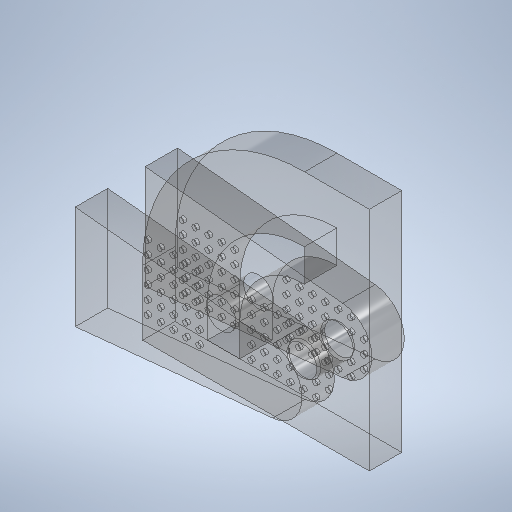
# Autodesk Inventor part: PruebadesoportesmecanismoV1
Saved by Autodesk Inventor 2025.2 (Build 292293000, 293)
## iProperties
Created: 2025-03-25
Part Number: PruebadesoportesmecanismoV1
Material: PVC, no plastificado
Document SubType Name: Modeling
Designer: braug
Density: 1.29 g/cm^3
Appearance: Agua Burbujas
Author: braug
## iProperties of the stored document Prueba de soportes mecanismo_3DPrint.ipt
Created: 2025-03-25
Part Number: Prueba de soportes mecanismo_3DPrint
Material: Genérico
Document SubType Name: Modeling
Designer: braug
Density: 1 g/cm^3
Appearance: Valor por defecto
Author: braug
Autodesk Inventor part; units mm, degrees
ref_plane "YZ Plane" through (0, 0, 0) normal (1, 0, 0) x (0, 1, 0)
ref_plane "XZ Plane" through (0, 0, 0) normal (0, 1, 0) x (-1, 0, 0)
ref_plane "XY Plane" through (0, 0, 0) normal (0, 0, 1) x (1, 0, 0)
sketch "Boceto1" plane through (0, 0, 0) normal (0, 0, 1) x (1, 0, 0)
  line L0 (-35, 0) -> (15, 0)
  line L1 (-20, 10) -> (-20, 0)
  arc A0 (-10, 20) -> (-20, 10) centre (-10, 10) ccw
  arc A1 (-10, 25) -> (-25, 10) centre (-10, 10) ccw
  line L2 (-25, 10) -> (-25, 0)
  arc A2 (-10, 35) -> (-35, 10) centre (-10, 10) ccw
  line L3 (-35, 10) -> (-35, 0)
  line L4 (-35, 0) -> (-10, 0)
  circle A3 centre (-10, 10) radius 2.5
  line L5 (-10, 20) -> (0, 20)
  line L6 (0, 20) -> (0, 21.1803)
  line L7 (0, 25) -> (-10, 25)
  line L8 (-10, 35) -> (0, 35)
  line L9 (0, 35) -> (0, 25)
  line L10 (0, 20) -> (0, 0)
  line L11 (0, 0) -> (-10, 0)
  line L12 (0, 25) -> (0, 20)
  line L13 (-10, 25) -> (-10, 20)
  line L14 (-20, 5) -> (-25, 5)
  point P0 (0, 0)
  dimension "d0" = 20
  dimension "d1" = 25
  dimension "d2" = 10
  dimension "d3" = 10
  dimension "d4" = 5
  dimension "d6" = 35
  constraints: 30 end point, 7 point on circle, 5 point on line, 4 centre point, 3 coincident, 3 collinear, 3 midpoint, 3 perpendicular, 3 tangent, 2 parallel, 1 horizontal
  measures "d0" distance of L5.start L11.end
  measures "d1" distance of L7.end L11.end
  measures "d2" distance of L3.start L0.start
  measures "d3" distance of L11.end A2.centre
  measures "d4" diameter of A3
  measures "d6" distance of L10.end L8.end
extrude "Extrusión1" add sketch "Boceto1" along normal mid plane 5 contours L3 A2 L8 L9 L7 A1 L2 L0 | L2 L14 L1 L0 | L1 A0 L5 L10 L0 | L7 L12 L6 L5 L13
sketch "Boceto2" plane through (0, 0, 2.5) normal (0, 0, 1) x (1, 0, 0)
  circle A0 centre (-10, 10) radius 2.3
  circle A1 centre (-22.5, 10) radius 2.3
  circle A2 centre (-10, 10) radius 2.5 projected
  point P0 (0, 0)
  dimension "d9" = 4.6
  dimension "d10" = 4.6
  constraints: 2 centre point
  measures "d9" diameter of A0
  measures "d10" diameter of A1
extrude "Extrusión2" add sketch "Boceto2" along normal blind 0.4 and the other way blind 5.4 contours A0 | A1
sketch "Boceto3" plane through (-10, 10, 2.9) normal (0, 0, 1) x (1, 0, 0)
  arc A0 (5, 0) -> (0.4927, 4.9757) centre (0, 0) ccw
  line L0 (-30, 0) -> (-30, 7.9951)
  line L1 (0.4927, 4.9757) -> (-30, 7.9951)
  line L2 (-30, 0) -> (-30, -7.9951)
  line L3 (0.4927, -4.9757) -> (-30, -7.9951)
  arc A1 (0.4927, -4.9757) -> (5, 0) centre (0, 0) ccw
  circle A2 centre (0, 0) radius 2.3 projected
  point P0 (10, -10)
  dimension "d15" = 10
  constraints: 8 end point, 4 point on circle, 2 centre point
  measures "d15" diameter of A0
extrude "Extrusión3" add sketch "Boceto3" along normal blind 5 contours A1 L3 L2 L0 L1 A0 | A2
sketch "Boceto4" plane through (-22.5, 10, -2.9) normal (0, 0, -1) x (-1, 0, 0)
  circle A0 centre (0, 0) radius 2.3 projected
  circle A1 centre (-12.5, 0) radius 2.3 projected
  line L0 (-12.9927, 4.9757) -> (17.5, 7.9951) projected
  arc A2 (-12.9927, 4.9757) -> (-12.9927, -4.9757) centre (-12.5, 0) ccw projected
  line L1 (17.5, -7.9951) -> (-12.9927, -4.9757) projected
  line L2 (17.5, 7.9951) -> (17.5, -7.9951) projected
  point P0 (-22.5, -10)
extrude "Extrusión4" add sketch "Boceto4" along normal blind 5 contours A0 | A1 | L0 L2 L1 A2
sketch "Boceto5" plane through (0, 0, -2.5) normal (0, 0, -1) x (-1, 0, 0)
  circle A0 centre (10, 10) radius 2.3 projected
  circle A1 centre (10, 10) radius 0.4
  line L0 (10, 10) -> (10, 1.6419)
  line L1 (10, 1.6419) -> (12.8355, 1.6419)
  circle A2 centre (10, 8) radius 0.4
  circle A3 centre (10, 6) radius 0.4
  circle A4 centre (12, 10) radius 0.4
  circle A5 centre (12, 8) radius 0.4
  circle A6 centre (12, 6) radius 0.4
  circle A7 centre (14, 10) radius 0.4
  circle A8 centre (14, 8) radius 0.4
  circle A9 centre (14, 6) radius 0.4
  circle A10 centre (16, 10) radius 0.4
  circle A11 centre (16, 8) radius 0.4
  circle A12 centre (16, 6) radius 0.4
  circle A13 centre (18, 10) radius 0.4
  circle A14 centre (18, 8) radius 0.4
  circle A15 centre (18, 6) radius 0.4
  circle A16 centre (20, 10) radius 0.4
  circle A17 centre (20, 8) radius 0.4
  circle A18 centre (20, 6) radius 0.4
  circle A19 centre (22, 10) radius 0.4
  circle A20 centre (22, 8) radius 0.4
  circle A21 centre (22, 6) radius 0.4
  circle A22 centre (24, 10) radius 0.4
  circle A23 centre (24, 8) radius 0.4
  circle A24 centre (24, 6) radius 0.4
  circle A25 centre (26, 10) radius 0.4
  circle A26 centre (26, 8) radius 0.4
  circle A27 centre (26, 6) radius 0.4
  circle A28 centre (28, 10) radius 0.4
  circle A29 centre (28, 8) radius 0.4
  circle A30 centre (28, 6) radius 0.4
  circle A31 centre (30, 10) radius 0.4
  circle A32 centre (30, 8) radius 0.4
  circle A33 centre (30, 6) radius 0.4
  circle A34 centre (32, 10) radius 0.4
  circle A35 centre (32, 8) radius 0.4
  circle A36 centre (32, 6) radius 0.4
  circle A37 centre (34, 10) radius 0.4
  circle A38 centre (34, 8) radius 0.4
  circle A39 centre (34, 6) radius 0.4
  circle A40 centre (36, 10) radius 0.4
  circle A41 centre (36, 8) radius 0.4
  circle A42 centre (36, 6) radius 0.4
  circle A43 centre (38, 10) radius 0.4
  circle A44 centre (38, 8) radius 0.4
  circle A45 centre (38, 6) radius 0.4
  circle A46 centre (10, 14) radius 0.4
  line L2 (10, 14) -> (10, 5.6419)
  circle A47 centre (10, 12) radius 0.4
  circle A48 centre (14, 14) radius 0.4
  circle A49 centre (14, 12) radius 0.4
  circle A50 centre (14, 10) radius 0.4
  circle A51 centre (12, 14) radius 0.4
  circle A52 centre (12, 12) radius 0.4
  circle A53 centre (12, 10) radius 0.4
  circle A54 centre (10, 10) radius 0.4
  circle A55 centre (16, 10) radius 0.4
  circle A56 centre (22, 14) radius 0.4
  circle A57 centre (22, 12) radius 0.4
  circle A58 centre (22, 10) radius 0.4
  circle A59 centre (24, 10) radius 0.4
  circle A60 centre (24, 12) radius 0.4
  circle A61 centre (24, 14) radius 0.4
  circle A62 centre (26, 10) radius 0.4
  circle A63 centre (26, 14) radius 0.4
  circle A64 centre (26, 12) radius 0.4
  circle A65 centre (28, 14) radius 0.4
  circle A66 centre (28, 12) radius 0.4
  circle A67 centre (28, 10) radius 0.4
  circle A68 centre (30, 10) radius 0.4
  circle A69 centre (30, 12) radius 0.4
  circle A70 centre (30, 14) radius 0.4
  circle A71 centre (32, 10) radius 0.4
  circle A72 centre (32, 12) radius 0.4
  circle A73 centre (32, 14) radius 0.4
  circle A74 centre (34, 14) radius 0.4
  circle A75 centre (34, 12) radius 0.4
  circle A76 centre (34, 10) radius 0.4
  circle A77 centre (36, 12) radius 0.4
  circle A78 centre (36, 10) radius 0.4
  circle A79 centre (36, 14) radius 0.4
  circle A80 centre (38, 10) radius 0.4
  circle A81 centre (38, 12) radius 0.4
  circle A82 centre (38, 14) radius 0.4
  circle A83 centre (16, 12) radius 0.4
  circle A84 centre (18, 12) radius 0.4
  circle A85 centre (18, 10) radius 0.4
  circle A86 centre (18, 14) radius 0.4
  circle A87 centre (20, 10) radius 0.4
  circle A88 centre (20, 12) radius 0.4
  circle A89 centre (20, 14) radius 0.4
  circle A90 centre (16, 14) radius 0.4
  circle A91 centre (8, 10) radius 0.4
  circle A92 centre (8, 8) radius 0.4
  circle A93 centre (8, 6) radius 0.4
  circle A94 centre (6, 10) radius 0.4
  circle A95 centre (6, 8) radius 0.4
  circle A96 centre (6, 6) radius 0.4
  circle A97 centre (8, 14) radius 0.4
  circle A98 centre (8, 12) radius 0.4
  circle A99 centre (8, 10) radius 0.4
  circle A100 centre (6, 14) radius 0.4
  circle A101 centre (6, 12) radius 0.4
  circle A102 centre (6, 10) radius 0.4
  circle A103 centre (10, 6) radius 0.4
  circle A104 centre (12, 6) radius 0.4
  circle A105 centre (14, 6) radius 0.4
  circle A106 centre (16, 6) radius 0.4
  circle A107 centre (18, 6) radius 0.4
  circle A108 centre (20, 6) radius 0.4
  circle A109 centre (22, 6) radius 0.4
  circle A110 centre (10, 4) radius 0.4
  circle A111 centre (12, 4) radius 0.4
  circle A112 centre (14, 4) radius 0.4
  circle A113 centre (16, 4) radius 0.4
  circle A114 centre (18, 4) radius 0.4
  circle A115 centre (20, 4) radius 0.4
  circle A116 centre (22, 4) radius 0.4
  circle A117 centre (24, 10) radius 0.4
  circle A118 centre (24, 8) radius 0.4
  circle A119 centre (24, 6) radius 0.4
  circle A120 centre (24, 4) radius 0.4
  circle A121 centre (26, 10) radius 0.4
  circle A122 centre (26, 8) radius 0.4
  circle A123 centre (26, 6) radius 0.4
  circle A124 centre (26, 4) radius 0.4
  circle A125 centre (28, 10) radius 0.4
  circle A126 centre (28, 8) radius 0.4
  circle A127 centre (28, 6) radius 0.4
  circle A128 centre (28, 4) radius 0.4
  circle A129 centre (30, 10) radius 0.4
  circle A130 centre (30, 8) radius 0.4
  circle A131 centre (30, 6) radius 0.4
  circle A132 centre (30, 4) radius 0.4
  circle A133 centre (32, 10) radius 0.4
  circle A134 centre (32, 8) radius 0.4
  circle A135 centre (32, 6) radius 0.4
  circle A136 centre (32, 4) radius 0.4
  circle A137 centre (34, 10) radius 0.4
  circle A138 centre (34, 8) radius 0.4
  circle A139 centre (34, 6) radius 0.4
  circle A140 centre (34, 4) radius 0.4
  circle A141 centre (36, 10) radius 0.4
  circle A142 centre (36, 8) radius 0.4
  circle A143 centre (36, 6) radius 0.4
  circle A144 centre (36, 4) radius 0.4
  point P0 (0, 0)
  dimension "d20" = 0.8
  dimension "d23" = 2
  dimension "d26" = 2
  dimension "d31" = 4
  dimension "d38" = 6
  constraints: 144 centre point, 6 end point, 3 vertical, 2 coincident, 2 horizontal, 1 collinear, 1 perpendicular, 226 other
  measures "d20" diameter of A1
  measures "d23" distance of A1.centre A2.centre
  measures "d26" distance of A1.centre A4.centre
  measures "d31" distance of A1.centre A46.centre
  measures "d38" distance of A7.centre A91.centre
extrude "Extrusión5" add sketch "Boceto5" along normal up to next contours A0 A4 | A0 A4 | A3 L0 | L0 A3 | A46 | A5 | A6 | A7 | A8 | A9 | A10 | A11 | A12 | A13 | A14 | A15 | A25 | A26 | A27 | A28 | A29 | A30 | A31 | A32 | A33 | A34 | A35 | A36 | A37 | A38 | A39 | A48 | A49 | A51 | A52 | A63 | A64 | A65 | A66 | A69 | A70 | A72 | A73 | A74 | A75 | A83 | A84 | A86 | A90 | A92 | A93 | A94 | A95 | A97 | A98 | A101 | A124 | A128 | A132 | A136 | A140
mirror "Simetría1" about plane through (0, 0, 0) normal (0, 0, 1) of "Extrusión5"
